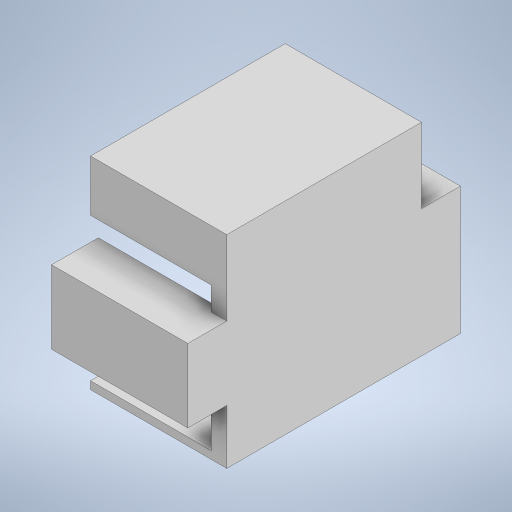
# Autodesk Inventor part: servoHolderBase
Saved by Autodesk Inventor 2024 (Build 280153000, 153)
## iProperties
Created: 2024-08-21
Part Number: servoHolderBase
Material: Generic
Document SubType Name: Modeling
Designer: omiye
Density: 1 g/cm^3
Appearance: Default
Author: omiye
Autodesk Inventor part; units mm, degrees
ref_plane "YZ Plane" through (0, 0, 0) normal (1, 0, 0) x (0, 1, 0)
ref_plane "XZ Plane" through (0, 0, 0) normal (0, 1, 0) x (-1, 0, 0)
ref_plane "XY Plane" through (0, 0, 0) normal (0, 0, 1) x (1, 0, 0)
sketch "Sketch1" plane through (0, 0, 0) normal (1, 0, 0) x (0, 1, 0)
  line L0 (-12, 12.25) -> (12, 12.25)
  line L1 (12, 12.25) -> (12, -12.25)
  line L2 (12, -12.25) -> (-12, -12.25)
  line L3 (-12, -12.25) -> (-12, 12.25)
  line L4 (-12, 12.25) -> (12, -12.25) construction
  line L5 (12, 12.25) -> (-12, -12.25) construction
  line L6 (-13, -13.25) -> (13, -13.25)
  line L7 (13, -13.25) -> (13, 13.25)
  line L8 (13, 13.25) -> (-13, 13.25)
  line L9 (-13, 13.25) -> (-13, -13.25)
  line L10 (-13, -13.25) -> (13, 13.25) construction
  line L11 (13, -13.25) -> (-13, 13.25) construction
  point P0 (0, 0)
  dimension "d0" = 24
  dimension "d1" = 24.5
  dimension "d2" = 26
  dimension "d3" = 26.5
  constraints: 24 end point, 4 midpoint, 4 parallel, 2 horizontal, 2 perpendicular
  measures "d0" distance of L1.end L2.end
  measures "d1" distance of L0.end L1.end
  measures "d2" distance of L8.end L7.end
  measures "d3" distance of L7.end L6.end
extrude "Extrusion1" add sketch "Sketch1" along normal blind 14.5
sketch "Sketch2" plane through (0, 13, 13.25) normal (0, 1, 0) x (1, 0, 0)
  line L0 (0, 26.5) -> (14.5, 26.5) projected
  line L1 (0, 0) -> (14.5, 0) projected
  line L2 (14.5, 26.5) -> (12.5, 26.5)
  line L3 (12.5, 26.5) -> (12.5, 0)
  line L4 (12.5, 0) -> (14.5, 0)
  line L5 (14.5, 0) -> (14.5, 26.5)
  point P0 (0, 13.25)
  dimension "d6" = 2
  constraints: 8 end point, 2 parallel, 1 horizontal, 1 perpendicular, 1 point on line
  measures "d6" distance of L4.end L3.end
extrude "Extrusion2" add sketch "Sketch2" against normal blind 26
sketch "Sketch3" plane through (0, 0, 0) normal (-1, 0, 0) x (0, 0, 1)
  point P0 (0, 0)
sketch "Sketch4" plane through (0, 0, 0) normal (-1, 0, 0) x (0, 0, 1)
  line L0 (13.25, -13) -> (-13.25, -13) projected
  line L1 (-13.25, 13) -> (13.25, 13)
  line L2 (13.25, 13) -> (13.25, -13)
  line L3 (13.25, -13) -> (-13.25, -13)
  line L4 (-13.25, -13) -> (-13.25, 13)
  line L5 (12.25, -12) -> (-12.25, -12) projected
  line L6 (-12.25, 12) -> (12.25, 12)
  line L7 (12.25, 12) -> (12.25, -12)
  line L8 (12.25, -12) -> (-12.25, -12)
  line L9 (-12.25, -12) -> (-12.25, 12)
  point P0 (0, 0)
  constraints: 16 end point, 4 parallel, 2 horizontal, 2 perpendicular
extrude "Extrusion3" add sketch "Sketch4" along normal blind 3
sketch "Sketch5" plane through (12.5, -12, 12.25) normal (-1, 0, 0) x (0, 0, 1)
  line L0 (-24.5, 24) -> (0, 24) projected
  line L1 (0, 24) -> (0, 0) projected
  line L2 (-24.5, 24) -> (0, 24)
  line L3 (0, 24) -> (0, 0)
  line L4 (0, 0) -> (-24.5, 0)
  line L5 (-24.5, 0) -> (-24.5, 24)
  line L6 (-24.5, 24) -> (-24.5, 12)
  line L7 (-24.5, 0) -> (-24.5, 24) projected
  line L8 (-0.5, 0) -> (-24, 0)
  line L9 (-24, 0) -> (-24, 24)
  line L10 (-24, 24) -> (-0.5, 24)
  line L11 (-0.5, 24) -> (-0.5, 0)
  line L12 (-0.5, 0) -> (-24, 24) construction
  line L13 (-24, 0) -> (-0.5, 24) construction
  point P0 (-12.25, 12)
  dimension "d11" = 23.5
  constraints: 22 end point, 4 parallel, 3 midpoint, 2 horizontal, 2 perpendicular, 1 point on line
  measures "d11" distance of L9.end L10.end
extrude "Extrusion4" add sketch "Sketch5" along normal blind 15.5 contours L0 L9 L4 L5 | L0 L1 L4 L11
sketch "Sketch6" plane through (-3, 0, 0) normal (-1, 0, 0) x (0, 0, 1)
  line L0 (13.25, 13) -> (-13.25, 13) projected
  line L1 (12.75, -13) -> (-12.75, -13)
  line L2 (-12.75, -13) -> (-12.75, 13)
  line L3 (-12.75, 13) -> (12.75, 13)
  line L4 (12.75, 13) -> (12.75, -13)
  line L5 (12.75, -13) -> (-12.75, 13) construction
  line L6 (-12.75, -13) -> (12.75, 13) construction
  line L7 (-13.25, 13) -> (13.25, 13) projected
  line L8 (-13.25, 13) -> (-12.5, 13)
  line L9 (-12.5, 13) -> (-12.5, -13)
  line L10 (-12.5, -13) -> (-13.25, -13)
  line L11 (-13.25, -13) -> (-13.25, 13)
  line L12 (13.2549, -13) -> (12.5049, -13)
  line L13 (12.5049, -13) -> (12.5049, 13)
  line L14 (12.5049, 13) -> (13.2549, 13)
  line L15 (13.2549, 13) -> (13.2549, -13)
  point P0 (0, 0)
  dimension "d14" = 25.5
  dimension "d15" = 0.75
  dimension "d16" = 0.75
  constraints: 28 end point, 6 parallel, 4 point on line, 3 horizontal, 3 perpendicular, 2 midpoint
  measures "d14" distance of L2.end L3.end
  measures "d15" distance of L9.end L10.end
  measures "d16" distance of L13.end L14.end
extrude "Extrusion5" cut sketch "Sketch6" against normal blind 18.25 contours L14 L15 L12 L4 L0 | L4 L1 L13 L0 | L9 L1 L2 L0 | L2 L10 L11 L0
sketch "Sketch7" plane through (-3, 0, 0) normal (-1, 0, 0) x (0, 0, 1)
  line L0 (-11.75, -12) -> (-11.75, 12) projected
  line L1 (11.75, -12) -> (-11.75, -12) projected
  line L2 (-11.75, 12) -> (-11.5, 12)
  line L3 (-11.5, 12) -> (-11.5, -12)
  line L4 (-11.5, -12) -> (-11.75, -12)
  line L5 (-11.75, -12) -> (-11.75, 12)
  line L6 (11.75, 12) -> (11.75, -12) projected
  line L7 (-11.75, 12) -> (11.75, 12) projected
  line L8 (11.75, -12) -> (11.5, -12)
  line L9 (11.5, -12) -> (11.5, 12)
  line L10 (11.5, 12) -> (11.75, 12)
  line L11 (11.75, 12) -> (11.75, -12)
  point P0 (0, 0)
  dimension "d19" = 0.25
  dimension "d20" = 0.25
  constraints: 16 end point, 4 parallel, 2 horizontal, 2 perpendicular, 2 point on line
  measures "d19" distance of L3.end L4.end
  measures "d20" distance of L9.end L10.end
extrude "Extrusion6" add sketch "Sketch7" against normal blind 17.25 contours L0 L2 L3 L1 | L9 L7 L6 L1
sketch "Sketch8" plane through (-3, -13, -12.5) normal (0, 0, -1) x (-1, 0, 0)
  line L0 (-17.5, 0) -> (0, 0) projected
  line L1 (0, 0) -> (0, 26) projected
  line L2 (-17.5, 0) -> (0, 0)
  line L3 (0, 0) -> (0, 15.4)
  line L4 (0, 15.4) -> (-17.5, 15.4)
  line L5 (-17.5, 15.4) -> (-17.5, 0)
  point P0 (-3, 13)
  dimension "d23" = 15.4
  constraints: 8 end point, 2 parallel, 1 horizontal, 1 perpendicular, 1 point on line
  measures "d23" distance of L3.end L2.end
extrude "Extrusion7" add sketch "Sketch8" along normal blind 5
sketch "Sketch9" plane through (14.5, 13, -12.5) normal (0, 0, -1) x (-1, 0, 0)
  line L0 (0, -10.6) -> (0, -26) projected
  line L1 (17.5, -25) -> (17.5, -1) projected
  line L2 (0, -10.6) -> (17.5, -10.6)
  line L3 (17.5, -10.6) -> (17.5, -7.6)
  line L4 (17.5, -7.6) -> (0, -7.6)
  line L5 (0, -7.6) -> (0, -10.6)
  line L6 (2, -1) -> (2, -25) projected
  line L7 (0, -10.6) -> (2, -10.6)
  line L8 (2, -10.6) -> (2, -7.6)
  line L9 (2, -7.6) -> (0, -7.6)
  line L10 (0, -7.6) -> (0, -10.6)
  point P0 (14.5, -13)
  dimension "d26" = 3
  constraints: 16 end point, 4 parallel, 3 point on line, 2 horizontal, 2 perpendicular
  measures "d26" distance of L3.end L2.end
extrude "Extrusion8" cut sketch "Sketch9" against normal blind 5 contours L2 L6 L4 L1
sketch "Sketch10" plane through (-3, -13, -17.5) normal (0, 0, -1) x (-1, 0, 0)
  line L0 (0, 15.4) -> (-17.5, 15.4) projected
  line L1 (0, 0) -> (0, 26) projected
  line L2 (-17.5, 15.4) -> (0, 15.4)
  line L3 (0, 15.4) -> (0, 16.4)
  line L4 (0, 16.4) -> (-17.5, 16.4)
  line L5 (-17.5, 16.4) -> (-17.5, 15.4)
  point P0 (-3, 13)
  dimension "d29" = 1
  constraints: 8 end point, 2 parallel, 1 horizontal, 1 perpendicular, 1 point on line
  measures "d29" distance of L3.end L2.end
extrude "Extrusion9" add sketch "Sketch10" against normal blind 6
sketch "Sketch11" plane through (14.5, 13, -12.5) normal (0, 0, -1) x (-1, 0, 0)
  line L0 (2, -9.6) -> (2, -7.6) projected
  line L1 (17.5, 0) -> (17.5, -7.6) projected
  line L2 (2, -7.6) -> (17.5, -7.6)
  line L3 (17.5, -7.6) -> (17.5, -6.6)
  line L4 (17.5, -6.6) -> (2, -6.6)
  line L5 (2, -6.6) -> (2, -7.6)
  point P0 (14.5, -13)
  dimension "d32" = 1
  constraints: 8 end point, 2 parallel, 1 horizontal, 1 perpendicular, 1 point on line
  measures "d32" distance of L3.end L2.end
extrude "Extrusion10" cut sketch "Sketch11" against normal blind 6
sketch "Sketch12" plane through (-3, -13, 12.5049) normal (0, 0, 1) x (1, 0, 0)
  line L0 (17.5, 0) -> (0, 0) projected
  line L1 (17.5, 0) -> (0, 0)
  line L2 (0, 0) -> (0, 7)
  line L3 (0, 7) -> (17.5, 7)
  line L4 (17.5, 7) -> (17.5, 0)
  line L5 (17.5, 16.4) -> (17.5, 0) projected
  line L6 (0, 7) -> (17.5, 7)
  line L7 (17.5, 7) -> (17.5, 16.4)
  line L8 (17.5, 16.4) -> (0, 16.4)
  line L9 (0, 16.4) -> (0, 7)
  point P0 (3, 13)
  dimension "d35" = 7
  constraints: 16 end point, 4 parallel, 2 horizontal, 2 perpendicular
  measures "d35" distance of L1.end L2.end
extrude "Extrusion11" add sketch "Sketch12" along normal blind 5 contours L3 L9 L8 L5
sketch "Sketch13" plane through (-3, 13, 12.5049) normal (0, 0, 1) x (1, 0, 0)
  line L0 (17.5, -9.6) -> (17.5, -26) projected
  line L1 (0, -1) -> (0, -25) projected
  line L2 (17.5, -9.6) -> (0, -9.6)
  line L3 (0, -9.6) -> (0, -6.6)
  line L4 (0, -6.6) -> (17.5, -6.6)
  line L5 (17.5, -6.6) -> (17.5, -9.6)
  line L6 (17.5, -6.6) -> (15.5, -6.6)
  line L7 (15.5, -6.6) -> (15.5, -9.6)
  line L8 (15.5, -9.6) -> (17.5, -9.6)
  line L9 (17.5, -9.6) -> (17.5, -6.6)
  point P0 (3, -13)
  dimension "d38" = 3
  dimension "d39" = 2
  constraints: 16 end point, 4 parallel, 2 horizontal, 2 perpendicular, 2 point on line
  measures "d38" distance of L2.end L3.end
  measures "d39" distance of L8.end L7.end
extrude "Extrusion12" cut sketch "Sketch13" against normal blind 5 contours L4 L7 L2 L1
sketch "Sketch14" plane through (-3, -13, 12.5049) normal (0, 0, 1) x (1, 0, 0)
  line L0 (0, 1) -> (15.5, 1) projected
  line L1 (15.5, 16.4) -> (15.5, 1) projected
  line L2 (0, 1) -> (15.5, 1)
  line L3 (15.5, 1) -> (15.5, 7)
  line L4 (15.5, 7) -> (0, 7)
  line L5 (0, 7) -> (0, 1)
  point P0 (3, 13)
  dimension "d42" = 6
  constraints: 8 end point, 2 parallel, 1 horizontal, 1 perpendicular, 1 point on line
  measures "d42" distance of L3.end L2.end
extrude "Extrusion13" cut sketch "Sketch14" against normal blind 5
body "Solid1"
